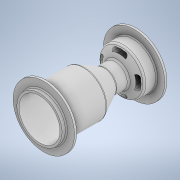
# Autodesk Inventor part: Trục mới
Saved by Autodesk Inventor 2022 (Build 260153000, 153)
## iProperties
Created: 2022-04-22
Part Number: Trục mới
Material: Generic
Document SubType Name: Modeling
Designer: duyne
Density: 1 g/cm^3
Appearance: Default
Author: duyne
Autodesk Inventor part; units mm, degrees
ref_plane "YZ Plane" through (0, 0, 0) normal (1, 0, 0) x (0, 1, 0)
ref_plane "XZ Plane" through (0, 0, 0) normal (0, 1, 0) x (-1, 0, 0)
ref_plane "XY Plane" through (0, 0, 0) normal (0, 0, 1) x (1, 0, 0)
sketch "Sketch1" plane through (0, 0, 0) normal (1, 0, 0) x (0, 1, 0)
  line L0 (10.5, 19.1401) -> (10.5, 17.1401)
  line L1 (10.5, 17.1401) -> (14.25, 17.1401)
  line L2 (14.25, 17.1401) -> (14.25, 16.1401)
  line L3 (14.25, 16.1401) -> (10.5, 16.1401)
  line L4 (10.5, 16.1401) -> (10.5, -1.2499)
  line L5 (10.3878, -1.7101) -> (5.6922, -10.7694)
  line L6 (5.58, -11.2296) -> (5.58, -16.0096)
  line L7 (6.1198, -16.8974) -> (9.9602, -18.888)
  line L8 (10.5, -19.7758) -> (10.5, -24.7758)
  line L9 (10.5, -24.7758) -> (14.25, -24.7758)
  line L10 (14.25, -24.7758) -> (14.25, -25.7758)
  line L11 (14.25, -25.7758) -> (10.5, -25.7758)
  line L12 (10.5, -25.7758) -> (10.5, -27.7758)
  line L13 (10.5, -27.7758) -> (0, -27.7758)
  line L14 (10.5, 19.1401) -> (0, 19.1401)
  line L15 (0, 28.5233) -> (0, -37.159) projected
  arc A0 (10.3878, -1.7101) -> (10.5, -1.2499) centre (9.5, -1.2499) ccw
  arc A1 (5.6922, -10.7694) -> (5.58, -11.2296) centre (6.58, -11.2296) ccw
  arc A2 (5.58, -16.0096) -> (6.1198, -16.8974) centre (6.58, -16.0096) ccw
  arc A3 (10.5, -19.7758) -> (9.9602, -18.888) centre (9.5, -19.7758) ccw
  point P0 (0, 0)
  point P1 (10.5, -1.4937)
  point P2 (5.58, -10.9859)
  dimension "d0" = 10.5
  dimension "d1" = 2
  dimension "d2" = 14.25
  dimension "d4" = 10.5
  dimension "d5" = 5.58
  dimension "d6" = 0
  dimension "d7" = 10.5
  dimension "d8" = 14.25
  dimension "d9" = 1
  dimension "d10" = 1
  dimension "d11" = 1
  dimension "d13" = 17.39
  dimension "d14" = 1
  dimension "d15" = 4.78
  dimension "d16" = 5
  dimension "d17" = 1
  dimension "d18" = 2
  constraints: 30 end point, 8 perpendicular, 8 point on circle, 8 point on line, 8 tangent, 4 centre point, 1 collinear, 1 equal radius, 1 horizontal, 1 parallel, 1 vertical
  measures "d0" distance of L0.start L14.end
  measures "d1" distance of L0.start L0.end
  measures "d2" distance from line of L15 L1.end
  measures "d4" distance between parallel lines of L15 L4
  measures "d5" distance from line of L15 point (5.58, -10.986)
  measures "d6" distance from line of L15 L13.end
  measures "d7" distance between parallel lines of L15 L8
  measures "d8" distance between parallel lines of L15 L10
  measures "d9" radius of A0
  measures "d10" radius of A1
  measures "d11" radius of A2
  measures "d13" distance of L3.end L4.end
  measures "d14" distance of L1.end L2.end
  measures "d15" distance of L6.start L6.end
  measures "d16" distance of L8.start L8.end
  measures "d17" distance of L9.end L10.end
  measures "d18" distance of L11.end L12.end
revolve "Revolution1" add sketch "Sketch1" angle 360 about axis through (0, 0, 0) along (0, 0, -1)
sketch "Sketch6" plane through (0, 0, -27.7758) normal (0, 0, -1) x (-1, 0, 0)
  circle A0 centre (0, 0) radius 4.5
  dimension "d19" = 9
  constraints: 1 centre point, 1 coincident
  measures "d19" diameter of A0
extrude "Extrusion1" cut sketch "Sketch6" against normal blind 85.725
sketch "Sketch7" plane through (0, 0, 19.1401) normal (0, 0, 1) x (1, 0, 0)
  circle A0 centre (0, 0) radius 9.5
  dimension "d22" = 19
  constraints: 1 centre point, 1 coincident
  measures "d22" diameter of A0
extrude "Extrusion2" cut sketch "Sketch7" against normal blind 21.1125
sketch "Sketch8" plane through (0, 0, -27.7758) normal (0, 0, -1) x (-1, 0, 0)
  circle A0 centre (0, 0) radius 9.5
  dimension "d25" = 19
  constraints: 1 centre point, 1 coincident
  measures "d25" diameter of A0
extrude "Extrusion3" cut sketch "Sketch8" against normal blind 5
sketch "Sketch9" plane through (0, 0, -22.7758) normal (0, 0, -1) x (-1, 0, 0)
  circle A0 centre (0, 0) radius 5.5
  dimension "d28" = 11
  constraints: 1 centre point, 1 coincident
  measures "d28" diameter of A0
extrude "Extrusion4" add sketch "Sketch9" along normal blind 1.8
sketch "Sketch10" plane through (0, 0, -24.5758) normal (0, 0, -1) x (-1, 0, 0)
  circle A0 centre (0, 0) radius 4.5
  dimension "d31" = 9
  constraints: 1 centre point, 1 coincident
  measures "d31" diameter of A0
extrude "Extrusion5" cut sketch "Sketch10" against normal blind 19.491
sketch "Sketch11" plane through (0, 0, -22.7758) normal (0, 0, -1) x (-1, 0, 0)
  circle A0 centre (0, 0) radius 5.5 projected
  arc A1 (0, 5.5) -> (2.3061, 6.1198) centre (0.5248, 8.1473) ccw
  line L0 (2.3061, 6.1198) -> (3.0697, 7.2802)
  arc A2 (3.0697, 7.2802) -> (2.3061, 9.2056) centre (2.0133, 7.9754) ccw
  line L1 (2.3061, 9.2056) -> (0, 9.4677)
  circle A3 centre (0, 0) radius 9.9602 projected
  arc A4 (-2.3061, 6.1198) -> (0, 5.5) centre (-0.5248, 8.1473) ccw
  line L2 (-2.3061, 6.1198) -> (-3.0697, 7.2802)
  arc A5 (-2.3061, 9.2056) -> (-3.0697, 7.2802) centre (-2.0133, 7.9754) ccw
  line L3 (-2.3061, 9.2056) -> (0, 9.4677)
  point P0 (-0.7056, 5.4545)
  point P1 (0.7056, 5.4545)
  dimension "d34" = 1.2645
  constraints: 8 end point, 8 point on circle, 4 centre point, 1 tangent, 2 other
  measures "d34" radius of A2
extrude "Extrusion6" cut sketch "Sketch11" against normal blind 4.991 contours A0 A4 L2 A5 L3 L1 A2 L0 A1
pattern_circular "Circular Pattern1" count 4 over 360 about axis through (0, 0, -17.8927) along (0, 0, -1) of "Extrusion6"
fillet "Fillet1" radius 0.5 1 edges at (0, -10.5, 16.1401)
fillet "Fillet2" radius 0.5 1 edges at (0, -10.5, 17.1401)
fillet "Fillet3" radius 0.5 1 edges at (0, -10.5, -24.7758)
fillet "Fillet4" radius 0.5 1 edges at (0, -10.5, -25.7758)
body "Solid1"
